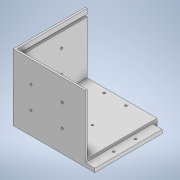
# Autodesk Inventor part: Quarter 2
Saved by Autodesk Inventor 2020.2 (Build 242310000, 310)
## iProperties
Created: 2020-01-17
Part Number: Quarter 2
Material: Generic
Document SubType Name: Modeling
Designer: ColinP
Density: 1 g/cm^3
Appearance: Default
Author: ColinP
Autodesk Inventor part; units mm, degrees
ref_plane "YZ Plane" through (0, 0, 0) normal (1, 0, 0) x (0, 1, 0)
ref_plane "XZ Plane" through (0, 0, 0) normal (0, 1, 0) x (-1, 0, 0)
ref_plane "XY Plane" through (0, 0, 0) normal (0, 0, 1) x (1, 0, 0)
sketch "Sketch1" plane through (0, 0, 0) normal (0, 1, 0) x (-1, 0, 0)
  line L0 (0, 0) -> (150, 0)
  line L1 (150, 0) -> (150, 150)
  line L2 (150, 150) -> (0, 150)
  line L3 (0, 150) -> (0, 0)
  dimension "d0" = 150
  dimension "d1" = 150
  constraints: 8 end point, 2 parallel, 1 horizontal, 1 perpendicular
  measures "d0" distance of L2.end L1.end
  measures "d1" distance of L1.end L0.end
extrude "Extrusion1" add sketch "Sketch1" along normal blind 10
sketch "Sketch2" plane through (0, 10, 0) normal (0, 1, 0) x (1, 0, 0)
  line L0 (0, 0) -> (-150, 0) projected
  line L1 (-150, 0) -> (-146, 0)
  line L2 (-146, 0) -> (-146, -146)
  line L3 (-146, -146) -> (0, -146)
  line L4 (0, -150) -> (0, 0) projected
  line L5 (-150, 0) -> (-150, -150) projected
  line L6 (-150, -150) -> (0, -150) projected
  line L7 (0, -150) -> (0, 0) projected
  line L8 (0, 0) -> (-150, 0) projected
  dimension "d4" = 4
  dimension "d5" = 146
  constraints: 6 end point, 2 perpendicular, 2 point on line
  measures "d4" distance of L0.end L1.end
  measures "d5" distance of L1.end L2.end
extrude "Extrusion2" add sketch "Sketch2" along normal blind 125 contours L2 L3 L4 L6 L5 L0
sketch "Sketch3" plane through (0, 0, 150) normal (1, 0, 0) x (0, 0, -1)
  line L0 (150, 0) -> (0, 0) projected
  line L1 (0, 0) -> (0, 5)
  line L2 (0, 0) -> (0, 135) projected
  line L3 (0, 5) -> (140, 5)
  line L4 (140, 5) -> (140, 0)
  line L5 (140, 0) -> (0, 0)
  dimension "d8" = 5
  dimension "d9" = 140
  dimension "d10" = 90
  constraints: 8 end point, 3 perpendicular, 1 point on line
  measures "d8" distance of L0.end L1.end
  measures "d9" distance of L1.end L3.end
  measures "d10" angle of L1 L3
extrude "Extrusion3" add sketch "Sketch3" along normal blind 20
sketch "Sketch4" plane through (0, 0, 0) normal (0, 0, -1) x (-1, 0, 0)
  line L0 (150, 0) -> (-20, 0) projected
  line L1 (150, 0) -> (150, 5)
  line L2 (150, 5) -> (10, 5)
  line L3 (10, 5) -> (10, 0)
  line L4 (10, 0) -> (150, 0)
  point P0 (0, 0)
  point P1 (10, 0)
  dimension "d13" = 5
  dimension "d14" = 140
  constraints: 8 end point, 3 perpendicular, 1 vertical
  measures "d13" distance of L0.start L1.end
  measures "d14" distance of L1.end L2.end
extrude "Extrusion4" cut sketch "Sketch4" against normal blind 20
sketch "Sketch5" plane through (0, 10, 146) normal (0, 0, -1) x (-1, 0, 0)
  line L0 (150, 125) -> (0, 125) projected
  line L1 (0, 125) -> (25, 125)
  line L2 (25, 125) -> (25, 85)
  line L3 (25, 85) -> (70, 85)
  line L4 (70, 85) -> (70, 28)
  line L5 (70, 28) -> (25, 28)
  line L6 (25, 28) -> (25, 85)
  line L7 (70, 85) -> (90, 85)
  line L8 (90, 85) -> (90, 28)
  line L9 (90, 28) -> (135, 28)
  line L10 (135, 28) -> (135, 85)
  line L11 (135, 85) -> (90, 85)
  line L12 (47.5, 85) -> (47.5, 80)
  line L13 (47.5, 80) -> (47.5, 33)
  line L14 (112.5, 85) -> (112.5, 80)
  line L15 (112.5, 80) -> (112.5, 33)
  point P0 (0, -10)
  dimension "d17" = 25
  dimension "d18" = 40
  dimension "d19" = 45
  dimension "d20" = 57
  dimension "d21" = 20
  dimension "d22" = 45
  dimension "d23" = 5
  dimension "d24" = 47
  dimension "d25" = 5
  dimension "d26" = 47
  constraints: 30 end point, 7 perpendicular, 7 point on line, 3 vertical, 2 midpoint, 1 collinear
  measures "d17" distance of L0.end L1.end
  measures "d18" distance of L1.end L2.end
  measures "d19" distance of L2.end L3.end
  measures "d20" distance of L3.end L4.end
  measures "d21" distance of L3.end L7.end
  measures "d22" distance of L8.end L9.end
  measures "d23" distance of L12.start L12.end
  measures "d24" distance of L12.end L13.end
  measures "d25" distance of L14.start L14.end
  measures "d26" distance of L14.end L15.end
hole "Hole1" at (-47.5, 90, 146) at (-112.5, 90, 146) at (-112.5, 43, 146) at (-47.5, 43, 146) direction (0, 0, 1) diameter 4.318 end through all
sketch "Sketch6" plane through (-146, 10, 146) normal (1, 0, 0) x (0, 0, -1)
  line L0 (0, 125) -> (146, 125) projected
  line L1 (0, 125) -> (70, 125)
  line L2 (70, 125) -> (70, 85)
  line L3 (70, 85) -> (115, 85)
  line L4 (115, 85) -> (115, 28)
  line L5 (115, 28) -> (70, 28)
  line L6 (70, 28) -> (70, 85)
  line L7 (92.5, 85) -> (92.5, 80)
  line L8 (92.5, 80) -> (92.5, 33)
  point P0 (146, -10)
  dimension "d34" = 70
  dimension "d35" = 40
  dimension "d36" = 45
  dimension "d37" = 57
  dimension "d38" = 5
  dimension "d39" = 47
  constraints: 16 end point, 4 perpendicular, 3 point on line, 1 collinear, 1 midpoint, 1 vertical
  measures "d34" distance of L0.start L1.end
  measures "d35" distance of L1.end L2.end
  measures "d36" distance of L2.end L3.end
  measures "d37" distance of L3.end L4.end
  measures "d38" distance of L7.start L7.end
  measures "d39" distance of L7.end L8.end
hole "Hole2" at (-146, 90, 53.5) at (-146, 43, 53.5) direction (-1, 0, 0) diameter 4.318 end through all
sketch "Sketch7" plane through (0, 0, 0) normal (0, -1, 0) x (1, 0, 0)
  line L0 (-150, 0) -> (-150, 150) projected
  line L1 (-150, 0) -> (-75, 0)
  line L2 (0, 0) -> (-146, 0) projected
  line L3 (-75, 0) -> (-75, 80)
  line L4 (-75, 80) -> (-55, 80)
  line L5 (-55, 80) -> (-95, 80)
  dimension "d47" = 75
  dimension "d48" = 80
  dimension "d49" = 20
  dimension "d50" = 40
  constraints: 8 end point, 2 perpendicular, 2 point on line
  measures "d47" distance of L0.start L1.end
  measures "d48" distance of L1.end L3.end
  measures "d49" distance of L3.end L4.end
  measures "d50" distance of L4.end L5.end
hole "Hole3" at (-95, 0, 80) at (-55, 0, 80) direction (0, 1, 0) diameter 4 end through all counterbore diameter 6 counterbore depth 3
sketch "Sketch8" plane through (-150, 0, 150) normal (-1, 0, 0) x (0, 0, 1)
  line L0 (-150, 10) -> (-150, 135) projected
  line L1 (-150, 135) -> (-150, 125)
  line L2 (-150, 125) -> (-4, 125)
  line L3 (-4, 10) -> (-4, 135) projected
  line L4 (-4, 125) -> (-4, 120)
  line L5 (-4, 120) -> (-150, 120)
  line L6 (-150, 125) -> (-150, 120)
  point P0 (-150, 0)
  dimension "d58" = 10
  dimension "d59" = 146
  dimension "d60" = 5
  constraints: 10 end point, 4 point on line, 1 collinear, 1 perpendicular
  measures "d58" distance of L0.end L1.end
  measures "d59" distance of L1.end L2.end
  measures "d60" distance of L2.end L4.end
extrude "Extrusion5" cut sketch "Sketch8" against normal blind 10
sketch "Sketch9" plane through (0, 10, 0) normal (0, 1, 0) x (1, 0, 0)
  line L0 (0, -10) -> (20, -10) projected
  line L1 (0, -10) -> (0, -55.3333)
  line L2 (0, -146) -> (0, 0) projected
  line L3 (0, -55.3333) -> (10, -55.3333)
  line L4 (10, -55.3333) -> (10, -100.6667)
  line L5 (-10, 0) -> (-10, -20) projected
  line L6 (-10, 0) -> (-55.3333, 0)
  line L7 (0, 0) -> (-146, 0) projected
  line L8 (-55.3333, 0) -> (-55.3333, -10)
  line L9 (-55.3333, -10) -> (-100.6667, -10)
  dimension "d63" = 45.3333
  dimension "d64" = 10
  dimension "d65" = 45.3333
  dimension "d66" = 45.3333
  dimension "d67" = 10
  dimension "d68" = 45.3333
  constraints: 12 end point, 4 perpendicular, 2 point on line
  measures "d63" distance of L0.start L1.end
  measures "d64" distance of L1.end L3.end
  measures "d65" distance of L3.end L4.end
  measures "d66" distance of L5.start L6.end
  measures "d67" distance of L6.end L8.end
  measures "d68" distance of L8.end L9.end
hole "Hole4" at (10, 10, 100.6667) at (10, 10, 55.3333) at (-55.3333, 10, 10) at (-100.6667, 10, 10) direction (0, -1, 0) diameter 4.318 end through all
sketch "Sketch10" plane through (0, 10, 0) normal (0, 1, 0) x (1, 0, 0)
  point P0 (0, 0)
sketch "Sketch11" plane through (0, 0, 0) normal (0, -1, 0) x (1, 0, 0)
  circle A0 centre (10, 100.6667) radius 2.159 projected
  circle A1 centre (10, 55.3333) radius 2.159 projected
  circle A2 centre (-95, 80) radius 3 projected
  circle A3 centre (-55, 80) radius 3 projected
  line L0 (-10, 20) -> (-10, 0) projected
  line L1 (0, 0) -> (-10, 0) projected
  line L2 (0, 10) -> (0, 0) projected
  line L3 (0, 10) -> (20, 10) projected
  line L4 (20, 150) -> (20, 10) projected
  line L5 (-150, 150) -> (20, 150) projected
  line L6 (-150, 20) -> (-150, 150) projected
  line L7 (-150, 20) -> (-10, 20) projected
extrude "Extrusion6" add sketch "Sketch11" along normal blind 3
sketch "Sketch12" plane through (-55, 3, 80) normal (0, -1, 0) x (1, 0, 0)
  circle A0 centre (0, 0) radius 3 projected
  circle A1 centre (0, 0) radius 2 projected
  circle A2 centre (-40, 0) radius 3 projected
  circle A3 centre (-40, 0) radius 2 projected
  point P0 (55, -80)
extrude "Extrusion7" add sketch "Sketch12" along normal blind 3
sketch "Sketch13" plane through (0, -3, 0) normal (0, -1, 0) x (1, 0, 0)
  circle A0 centre (10, 100.6667) radius 2.159 projected
  circle A1 centre (10, 55.3333) radius 2.159 projected
  point P0 (0, 0)
hole "Hole5" at (10, -3, 100.6667) at (10, -3, 55.3333) direction (0, 1, 0) diameter 4.318 end through all counterbore diameter 7.62 counterbore depth 5.08
body "Solid1"
